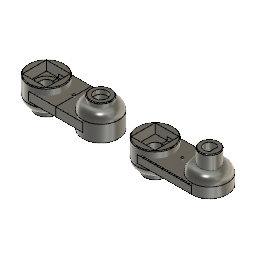
Links  big screw 11 v5 (Autodesk Fusion 360 design; units mm, degrees)
Autodesk Fusion 360 part; units mm, degrees
note: some values were not read from the file. Chosen so that the rebuilt part matches the saved one: which bodies a step acts on; which face or edge a step refers to. Set by a fixed rule: which sketch regions a step uses.
sketch "passive link sketch" plane through (0, 0, 0) normal (0, 0, 1) x (1, 0, 0) in component "PassiveLinkComponent"
  line L0 (-15.9748, 8.25) -> (-15.9748, -8.25) construction
  line L1 (15.9748, -8.25) -> (15.9748, 8.25) construction
  line L2 (15.9748, 8.25) -> (-15.9748, -8.25) construction
  line L3 (-15.9748, 8.25) -> (15.9748, -8.25) construction
  circle A0 centre (12.5, 0) radius 4.9
  circle A1 centre (12.5, 0) radius 2.975
  circle A2 centre (12.5, 0) radius 8.25
  line L4 (0, 8.25) -> (0, -15)
  line L5 (12.5, 8.25) -> (0, 8.25)
  line L6 (0, -8.25) -> (12.5, -8.25)
  line L7 (12.5, -8.25) -> (12.5, 8.25)
  line L8 (12.5, 8.25) -> (-12.5, -8.25) construction
  line L9 (-12.5, 8.25) -> (12.5, -8.25) construction
  line L10 (15.9748, 8.25) -> (0, 8.25) construction
  line L11 (-12.5, 8.25) -> (-15.9748, 8.25) construction
  line L12 (-15.9748, -8.25) -> (-12.5, -8.25) construction
  line L13 (0, -8.25) -> (15.9748, -8.25) construction
  line L14 (0, -8.25) -> (-15.9748, -8.25) construction
  line L15 (-12.5, -8.25) -> (-12.5, 8.25)
  line L16 (-15.9748, 8.25) -> (0, 8.25) construction
  circle A3 centre (-12.5, 0) radius 8.25
  circle A4 centre (-12.5, 0) radius 2.975
  circle A5 centre (-12.5, 0) radius 4.9
  line L17 (0, -8.25) -> (-12.5, -8.25)
  line L18 (-12.5, 8.25) -> (0, 8.25)
  line L19 (-7, 5.5) -> (-18, 5.5)
  line L20 (-18, 5.5) -> (-18, -5.5)
  line L21 (-18, -5.5) -> (-7, -5.5)
  line L22 (-7, -5.5) -> (-7, 5.5)
  line L23 (-7, 5.5) -> (-18, -5.5) construction
  line L24 (-18, 5.5) -> (-7, -5.5) construction
  circle A6 centre (0, 0) radius 0.6
  point P0 (-12.5, 0)
  dimension "d2" = 16.5
  dimension "d3" = 9.8
  dimension "d4" = 5.95
  dimension "d5" = 16.5
  dimension "d6" = 12.5
  dimension "d7" = 25
  dimension "d281" = 11
  dimension "d282" = 11
  dimension "d296" = 1.2
  constraint horizontal L10
  constraint perpendicular L0 L10
  constraint parallel L10 L12
  constraint parallel L0 L1
  constraint coincident L2 A6.centre
  constraint coincident L3 A6.centre
  constraint coincident A6.centre origin
  constraint concentric A0 A1
  constraint concentric A0 A2
  constraint perpendicular L4 L12
  constraint horizontal A6.centre A0.centre
  constraint horizontal L5
  constraint parallel L5 L6
  constraint coincident A2 L5.start
  constraint coincident L8 A6.centre
  constraint coincident L9 A6.centre
  constraint collinear L10 L11
  constraint coincident L4 L6.start
  constraint collinear L12 L13
  constraint symmetric L1.end L4 L0.start
  constraint symmetric L1.start L4 L0.end
  constraint symmetric A0 L4 A5
  constraint symmetric A1 L4 A4
  constraint symmetric A2 L4 A3
  constraint symmetric L4 L5.start L9.start
  constraint symmetric L4 L6.end L8.end
  constraint symmetric L4 L5.end L10.end
  constraint symmetric L4 L6.start L13.start
  constraint perpendicular L15 L18
  constraint coincident L4 A6.centre
  constraint horizontal L19
  constraint perpendicular L19 L20
  constraint parallel L19 L21
  constraint parallel L20 L22
  constraint coincident L23 P0
  constraint coincident L24 P0
  constraint coincident P0 A3.centre
  measures "d2" distance of L0.start L0.end
  measures "d3" diameter of A0
  measures "d4" diameter of A1
  measures "d5" diameter of A2
  measures "d6" distance of A6.centre A0.centre
  measures "d7" distance of L8.end L6.end
  measures "d281" distance of L20.end L21.end
  measures "d282" distance of L19.end L20.end
  measures "d296" diameter of A6
extrude "base" add sketch "passive link sketch" along normal mid plane 4 contours L4 A3 L17 L18 A6 | L4 A6 | L15 A3 L19 L21 L22 | L15 A5 L19 L21 L22 | L15 A4 A5 picked at (-0.1127, -0.1652) picked at (-12.2676, 4.2417) makes body 1 in component "PassiveLinkComponent"
extrude "l  big cyl" add sketch "passive link sketch" along normal blind 4.8 and the other way blind 7 separate body contours L15 A3 L19 L21 L22 | L15 A3 L19 L20 L21 | L15 A5 L19 L21 L22 | L15 A5 L19 L20 L21 | L15 A4 A5 | L15 A4 A5 makes body 2 in component "PassiveLinkComponent"
fillet "Fillet13" radius 4 1 edges at (-20.1917, 2.9833, -7) on bodies 2 in component "PassiveLinkComponent"
fillet "Fillet9" radius 0.3 1 edges at (-20.1917, -2.9833, 4.8) on bodies 2 in component "PassiveLinkComponent"
extrude "Extrude8" add sketch "passive link sketch" along normal blind 4.8 and the other way blind 9 separate body contours L15 A4 A5 | L15 A4 A5 makes body 3 in component "PassiveLinkComponent"
extrude "Extrude17" cut sketch "passive link sketch" along normal blind 4.4 from surface at 0.4 contours L15 A5 L19 L21 L22 | L15 A5 L19 L20 L21 | L15 A4 A5 | L15 A4 A5 | L15 A4 | L15 A4 bodies 1 2 3 in component "PassiveLinkComponent"
mirror "Mirror1" about plane through (0, 0, 0) normal (1, 0, 0) of bodies 2 1 3 makes body 4 at (3.1778, -0.0741, -2) makes body 5 at (4.291, 0.8214, -0.5) makes body 6 at (7.6243, 0.4879, -2.7333) in component "PassiveLinkComponent"
mirror "Mirror2" about plane through (0, 0, 0) normal (0, 0, 1) of bodies 6 5 4 makes body 7 at (7.6243, 0.4879, 2.7333) makes body 8 at (3.1778, -0.0741, 2) makes body 9 at (4.291, 0.8214, 0.5) in component "PassiveLinkComponent"
delete_body "RemoveBody3" bodies 5 in component "PassiveLinkComponent"
delete_body "RemoveBody4" bodies 6 in component "PassiveLinkComponent"
delete_body "RemoveBody5" bodies 4 in component "PassiveLinkComponent"
extrude "Extrude1" add sketch "passive link sketch" along normal blind 2.7 separate body contours L4 A6 | L4 A6 makes body 10 in component "PassiveLinkComponent"
move_face "OffsetFaces1" offset 0.3 1 faces at (-8.271, -0.3912, -9) on bodies 3 in component "PassiveLinkComponent"
fillet "Fillet14" radius 0.3 1 edges at (-17.4, 0, -9.3) on bodies 3 in component "PassiveLinkComponent"
fillet "Fillet1" radius 0.3 1 edges at (17.0684, 1.7719, 9) on bodies 7 in component "PassiveLinkComponent"
sketch "motorLinkSketch" plane through (0, 0, 0) normal (0, 0, 1) x (-1, 0, 0) in component "MotorLinkComponent"
  line L0 (12.5, -8.25) -> (12.5, 8.25)
  line L1 (0, 8) -> (0, -15) construction
  circle A0 centre (12.5, 0) radius 8.25
  circle A1 centre (12.5, 0) radius 2.975
  circle A2 centre (12.5, 0) radius 4.9
  circle A3 centre (-12.5, 0) radius 2.6
  circle A4 centre (-12.5, 0) radius 8.25
  line L2 (12.5, 8.25) -> (-12.5, 8.25)
  line L3 (12.5, -8.25) -> (-12.5, -8.25)
  line L4 (-14.4, -1.7748) -> (-14.4, 1.7748)
  line L5 (-12.5, -8.25) -> (-12.5, 8.25)
  line L6 (-9.9, -3.9402) -> (-9.9, 0.0066) construction
  circle A5 centre (-12.5, 0) radius 4.5
  line L7 (18, 5.5) -> (7, 5.5)
  line L8 (7, 5.5) -> (7, -5.5)
  line L9 (7, -5.5) -> (18, -5.5)
  line L10 (18, -5.5) -> (18, 5.5)
  line L11 (18, 5.5) -> (7, -5.5) construction
  line L12 (7, 5.5) -> (18, -5.5) construction
  circle A6 centre (0, 0) radius 0.5
  point P0 (-12.5, 0.7805)
  point P1 (12.5, 0)
  dimension "d215" = 9.8
  dimension "d216" = 5.95
  dimension "d217" = 16.5
  dimension "d218" = 12.5
  dimension "d222" = 16.5
  dimension "d223" = 5.2
  dimension "d261" = 25
  dimension "d262" = 4.5
  dimension "d269" = 9
  dimension "d277" = 1.9
  dimension "d279" = 11
  dimension "d280" = 11
  dimension "d299" = 1
  constraint coincident A6.centre origin
  constraint concentric A1 A2
  constraint concentric A0 A2
  constraint horizontal A6.centre A0.centre
  constraint coincident L0.end A0
  constraint coincident A6.centre L1
  constraint coincident A4 L2.end
  constraint tangent A4 L2
  constraint perpendicular L0 L2
  constraint coincident A4 L3.end
  constraint tangent A4 L3
  constraint perpendicular L0 L3
  constraint horizontal L3
  constraint coincident A3 L4.end
  constraint vertical L4
  constraint perpendicular L2 L5
  constraint coincident A3.centre L5
  constraint coincident A3 L4.start
  constraint concentric A3 A4
  constraint vertical L6
  constraint tangent A3 L6
  constraint concentric A3 A5
  constraint horizontal L7
  constraint perpendicular L7 L8
  constraint parallel L7 L9
  constraint parallel L8 L10
  constraint coincident L11 P1
  constraint coincident L12 P1
  constraint coincident P1 A0.centre
  measures "d215" diameter of A2
  measures "d216" diameter of A1
  measures "d217" diameter of A0
  measures "d218" distance of A6.centre A0.centre
  measures "d222" diameter of A4
  measures "d223" diameter of A3
  measures "d261" distance of P1 A3.centre
  measures "d262" distance of L4 L6.start
  measures "d269" diameter of A5
  measures "d277" distance of A3.centre L4
  measures "d279" distance of L8.end L9.end
  measures "d280" distance of L7.end L8.end
  measures "d299" diameter of A6
extrude "Extrude19" add sketch "motorLinkSketch" along normal blind 2.7 separate body contours A6 makes body 11 in component "MotorLinkComponent"
extrude "Extrude13" add sketch "motorLinkSketch" along normal mid plane 4 separate body contours L0 A0 L7 L8 L9 | A0 A4 L2 L3 | L0 A2 L7 L8 L9 | A4 L5 A5 | L0 A1 A2 | A3 L5 A5 | A6 picked at (-5.5433, -0.6048) picked at (12.2566, -4.2401) picked at (-8.6574, -0.3368) makes body 12 in component "MotorLinkComponent"
extrude "Extrude14" add sketch "motorLinkSketch" along normal blind 4.8 and the other way blind 7 separate body contours L0 A0 L7 L8 L9 | L0 A0 L7 L9 L10 | L0 A2 L7 L8 L9 | L0 A2 L7 L9 L10 | L0 A1 A2 | L0 A1 A2 makes body 13 in component "MotorLinkComponent"
extrude "Extrude17'" cut sketch "motorLinkSketch" along normal blind 4.4 from surface at 0.4 contours L0 A2 L7 L8 L9 | L0 A2 L7 L9 L10 | L0 A1 A2 | L0 A1 A2 | L0 A1 | L0 A1 bodies 12 13 in component "MotorLinkComponent"
extrude "Extrude15" add sketch "motorLinkSketch" along normal blind -4.8 and the other way blind 9.3 contours L0 A1 A2 | L0 A1 A2 bodies 13 in component "MotorLinkComponent"
fillet "Fillet15" radius 0.3 1 edges at (-7.9316, -1.7719, -9.3) on bodies 13 in component "MotorLinkComponent"
fillet "Fillet5" radius 4 1 edges at (-4.8083, -2.9833, -7) on bodies 13 in component "MotorLinkComponent"
fillet "Fillet7" radius 0.3 1 edges at (-4.8083, 2.9833, 4.8) on bodies 13 in component "MotorLinkComponent"
extrude "Extrude16" add sketch "motorLinkSketch" along normal blind 7 and the other way blind 2 separate body contours A4 L5 A5 | A4 L5 A5 | A3 L5 A5 | A3 L5 A5 | A3 L4 makes body 14 in component "MotorLinkComponent"
extrude "Extrude18" add sketch "motorLinkSketch" along normal blind 13.2 separate body contours A3 L5 A5 | A3 L5 A5 | A3 L4 makes body 15 in component "MotorLinkComponent"
fillet "Fillet13'" radius 0.3 1 faces at (12.7243, 4.4944, 8.8) on bodies 15 in component "MotorLinkComponent"
fillet "Fillet14'" radius 4 1 edges at (20.1917, 2.9833, 7) on bodies 14 in component "MotorLinkComponent"
fillet "Fillet9'" radius 0.3 3 edges at (0, 8.25, -2) (20.1917, -2.9833, -2) (0, -8.25, -2) on bodies 12 14 in component "MotorLinkComponent"
fillet "Fillet10" radius 0.3 1 edges at (0, 8.25, 2) on bodies 12 in component "MotorLinkComponent"
fillet "Fillet11" radius 0.3 1 edges at (0, -8.25, 2) on bodies 12 in component "MotorLinkComponent"
fillet "Fillet12" radius 0.3 2 edges at (9.9, 0, 7) (14.4, 0, 7) on bodies 14 in component "MotorLinkComponent"
box "BoxPrimitive1" add length 4 width 25 height 8 placed x (0, 1, 0) y (-1, 0, 0) z (0, 0, 1) at (25, 0, 0) separate body makes body 16 in component "adjustment spacer"
move_body "Move1" bodies 16 to x (1, 0, 0) y (0, 1, 0) z (0, 0, 1) at (0, 33.9, 0) in component "adjustment spacer"
component "PassiveLinkComponent" placed x (1, 0, 0) y (0, 1, 0) z (0, 0, 1) at (0, 0, 0)
component "MotorLinkComponent" placed x (1, 0, 0) y (0, 1, 0) z (0, 0, 1) at (50, 0, 0)
component "adjustment spacer" placed x (1, 0, 0) y (0, 1, 0) z (0, 0, 1) at (0, 0, 0)
equation "d2 = bigBarrelDiam"
equation "d3 = restShoulderDiam"
equation "d4 = screwHoleDiam"
equation "d5 = bigBarrelDiam"
equation "d8 = rectHeight / 2"
equation "d16 = nutSideHeight"
equation "d22 = nutSideHeight"
equation "d24 = nipScrewSideHeight"
equation "d25 = 0.0 °"
equation "d52 = screwSideBarrelHeight"
equation "d53 = 0.0 °"
equation "rectHeight = 4 mm"
equation "bigBarrelDiam = 16.5 mm"
equation "screwHoleDiam = 5.95 mm"
equation "shaftDiameter = 5.2 mm"
equation "rectLen = 25 mm"
equation "d134 = nutHeight"
equation "d151 = smallFillet"
equation "restShoulderDiam = 9.8 mm"
equation "nutSideHeight = 4.8 mm"
equation "nipScrewSideHeight = 9 mm"
equation "d206 = bigFillet"
equation "nutHeight = 4.4 mm"
equation "d209 = smallFillet"
equation "shaftNotchDelta = 4.5 mm"
equation "d215 = restShoulderDiam"
equation "d216 = screwHoleDiam"
equation "d217 = bigBarrelDiam"
equation "d218 = rectLen / 2"
equation "d222 = bigBarrelDiam"
equation "d223 = shaftDiameter"
equation "d228 = rectHeight / 2"
equation "d230 = nutSideHeight"
equation "d232 = screwSideBarrelHeight"
equation "d233 = 0.0 °"
equation "d234 = -nutSideHeight"
equation "d236 = nipScrewSideHeight + printerCompensationForHeight"
equation "d237 = 0.0 °"
equation "bigFillet = 4 mm"
equation "smallFillet = 0.3 mm"
equation "d241 = bigFillet"
equation "d245 = smallFillet"
equation "shaftHeight = 13.2 mm"
equation "d247 = screwSideBarrelHeight"
equation "d249 = rectHeight / 2"
equation "d250 = 0.0 °"
equation "d254 = smallFillet"
equation "d256 = smallFillet"
equation "d258 = smallFillet"
equation "d260 = smallFillet"
equation "d261 = rectLen"
equation "d262 = shaftNotchDelta"
equation "nutRectangularDimesion = 11 mm"
equation "d266 = nutHeight"
equation "screwSideBarrelHeight = nipScrewSideHeight - 2 mm"
equation "d269 = shaftSmallCilinderDiam"
equation "shaftSmallCilinderDiam = 9 mm"
equation "d271 = shaftHeight"
equation "d274 = smallFillet"
equation "d276 = bigFillet"
equation "d279 = nutRectangularDimesion"
equation "d280 = nutRectangularDimesion"
equation "d281 = nutRectangularDimesion"
equation "d282 = nutRectangularDimesion"
equation "d283 = nutSideHeight - nutHeight"
equation "d284 = nutSideHeight - nutHeight"
equation "printerCompensationForHeight = 0.3 mm"
equation "d291 = printerCompensationForHeight"
equation "d293 = smallFillet"
equation "d295 = smallFillet"
equation "d297 = rectHeight / 2 + 0.7 mm"
equation "d300 = rectHeight / 2 + 0.7 mm"
named bodies: "screwHole", "cuboid", "link part", "cuboid (1)", "big barrel (1)", "screwHole (1)", "screwHole (1) (1)", "cuboid (1) (1)", "big barrel (1) (1)", "barrel", "shaftSmallCilinder", "spacer tool", "bump for marking top side", "bamp for marking top side"
